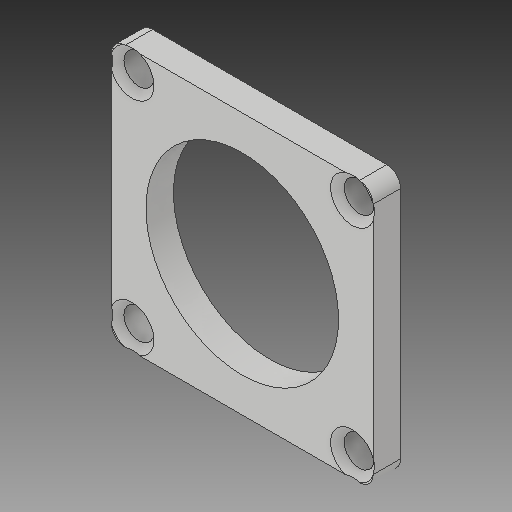
# Autodesk Inventor part: 20_Cube_Insert_Sample_clamp_magnetic
Saved by Autodesk Inventor 2019 (Build 230136000, 136)
## iProperties
Created: 2020-05-20
Part Number: 20_Cube_Insert_Sample_clamp_magnetic
Material: Generic
Document SubType Name: Modeling
Designer: B
Density: 1 g/cm^3
Appearance: Default
Author: B
Autodesk Inventor part; units mm, degrees
ref_plane "YZ Plane" through (0, 0, 0) normal (1, 0, 0) x (0, 1, 0)
ref_plane "XZ Plane" through (0, 0, 0) normal (0, 1, 0) x (-1, 0, 0)
sketch "Sketch1" plane through (0, 0, 0) normal (0, 0, 1) x (1, 0, 0)
  circle A0 centre (16.0203, -16.0203) radius 2.75 construction
  circle A1 centre (-16.0203, 16.0203) radius 2.75 construction
  circle A2 centre (16.0203, 16.0203) radius 2.75 construction
  circle A3 centre (-16.0203, -16.0203) radius 2.75 construction
  circle A4 centre (0, 0) radius 12.5 construction
  line L0 (17.0203, -19.0203) -> (-17.0203, -19.0203)
  line L1 (-19.0203, -17.0203) -> (-19.0203, 17.0203)
  line L2 (-17.0203, 19.0203) -> (17.0203, 19.0203)
  line L3 (19.0203, 17.0203) -> (19.0203, -17.0203)
  line L4 (19.0203, -19.0203) -> (-19.0203, 19.0203) construction
  line L5 (-19.0203, -19.0203) -> (19.0203, 19.0203) construction
  arc A5 (-17.0203, 19.0203) -> (-19.0203, 17.0203) centre (-17.0203, 17.0203) ccw
  arc A6 (-19.0203, -17.0203) -> (-17.0203, -19.0203) centre (-17.0203, -17.0203) ccw
  arc A7 (17.0203, -19.0203) -> (19.0203, -17.0203) centre (17.0203, -17.0203) ccw
  arc A8 (19.0203, 17.0203) -> (17.0203, 19.0203) centre (17.0203, 17.0203) ccw
  circle A9 centre (0, 0) radius 14
  line L6 (16.9, 24.9006) -> (-16.9, 24.9006) projected
  line L7 (-16.9, 21.2821) -> (-16.9, 24.9006) projected
  line L8 (-21.2821, 16.9) -> (-16.9, 21.2821) projected
  line L9 (-24.9006, 16.9) -> (-21.2821, 16.9) projected
  line L10 (-24.9006, -16.9) -> (-24.9006, 16.9) projected
  line L11 (-21.2821, -16.9) -> (-24.9006, -16.9) projected
  line L12 (-16.9, -21.2821) -> (-21.2821, -16.9) projected
  line L13 (-16.9, -24.9006) -> (-16.9, -21.2821) projected
  line L14 (16.9, -24.9006) -> (-16.9, -24.9006) projected
  line L15 (16.9, -24.9006) -> (16.9, -21.2821) projected
  line L16 (16.9, -21.2821) -> (21.2821, -16.9) projected
  line L17 (21.2821, -16.9) -> (24.9006, -16.9) projected
  line L18 (24.9006, -16.9) -> (24.9006, -16.8) projected
  line L19 (24.9006, -16.8) -> (24.9006, 16.9) projected
  line L20 (24.9006, 16.9) -> (21.2821, 16.9) projected
  line L21 (21.2821, 16.9) -> (16.9, 21.2821) projected
  line L22 (16.9, 21.2821) -> (16.9, 24.9006) projected
  point P0 (16.8, 24.9006)
  point P1 (-16.8, 24.9006)
  point P2 (-24.9006, 16.8)
  point P3 (-24.9006, -16.8)
  point P4 (-16.8, -24.9006)
  point P5 (16.8, -24.9006)
  point P6 (24.9006, 16.8)
  dimension "d0" = 2
  dimension "d1" = 28
  constraints: 12 end point, 8 point on circle, 8 point on line, 8 tangent, 5 centre point, 3 equal radius, 2 midpoint, 2 parallel, 1 coincident, 1 horizontal, 1 perpendicular
  measures "d0" radius of A5
  measures "d1" diameter of A9
extrude "Extrusion1" add sketch "Sketch1" along normal blind 4 contours L0 A6 L1 A5 L2 A8 L3 A7
ref_plane "Work Plane1" through (-17.0203, 16.0203, 0) normal (0, 1, 0) x (1, 0, 0)
sketch "Sketch2" plane through (-17.0203, 16.0203, 0) normal (0, 1, 0) x (1, 0, 0)
  line L0 (3.0203, 0) -> (31.0203, 0) construction
  line L1 (0, 0) -> (-2, 0) construction
  line L2 (34.0406, 0) -> (0, 0) construction
  line L3 (36.0406, 0) -> (34.0406, 0) construction
  line L4 (34.0406, 0) -> (36.0406, 0) construction
  line L5 (0, 0) -> (34.0406, 0) construction
  line L6 (-2, 0) -> (0, 0) construction
  line L7 (31.0203, -4) -> (3.0203, -4) construction
  line L8 (-2, -4) -> (0, -4) construction
  line L9 (0, -4) -> (34.0406, -4) construction
  line L10 (34.0406, -4) -> (36.0406, -4) construction
  line L11 (36.0406, -4) -> (34.0406, -4) construction
  line L12 (34.0406, -4) -> (0, -4) construction
  line L13 (0, -4) -> (-2, -4) construction
  line L14 (33.8203, 0) -> (0.2203, 0) construction
  line L15 (33.0406, 0) -> (33.0406, -4) construction
  arc A0 (33.0406, -4.15) -> (33.0406, 1.15) centre (33.0406, -1.5) ccw
  line L16 (35.2252, -3) -> (36.2252, -4)
  line L17 (33.0406, -1.5) -> (35.6906, -1.5) construction
  line L18 (36.2252, -4) -> (33.0406, -4)
  line L19 (0, -4) -> (34.0406, -4) construction
  line L20 (33.0406, -4) -> (33.0406, 1.15)
  line L21 (36.0406, 0) -> (36.0406, -4) projected
  point P0 (17.0203, 0)
  dimension "d4" = 2.65
  dimension "d5" = 2.5
  dimension "d7" = 135
  dimension "d8" = 1.5
  dimension "d14" = 3
  constraints: 10 end point, 5 point on line, 4 point on circle, 2 vertical, 1 centre point, 1 collinear
  measures "d4" radius of A0
  measures "d5" distance from line of L9 L17.start
  measures "d7" angle of L11 L16
  measures "d8" vertical distance of L17.start L16.start
  measures "d14" distance between parallel lines of L21 L15
revolve "Revolution1" cut sketch "Sketch2" angle 360 about axis through (16.0203, 16.0203, 4) along (0, 0, -1)
pattern_circular "Circular Pattern1" count 4 over 360 about axis through (0, 0, -10) along (0, 0, 1) of "Revolution1"
body "Solid1"
